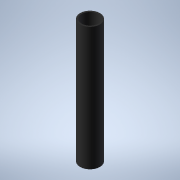
# Autodesk Inventor part: BZB-PDOWN
Saved by Autodesk Inventor 2021 (Build 250183000, 183)
## iProperties
Created: 2025-06-23
Part Number: BZB-PDOWN
Material: Generic
Catalog Web Link: www.cadenas.de
Description: base stand BZB-Accessories
Vendor: RNA
Document SubType Name: Modeling
Designer: psAdmin
Manufacturer: RNA
Mass: 179.196 g
Surface Area: 907.543 cm^2
Volume: 179.196 cm^3
Density: 1 g/cm^3
Appearance: PSOLRGB-175-175-175
Category: PARTsolutions
Company: RNA
Title: BZB-PDOWN
Author: Cadenas PARTsolutions
Comments: Accessories
PSOL_IDENT_0: {$CADENAS_DATA/23d-libs/rna/bunker/zubehoer/parts/bzb_profil_down.prj},166 {VTYP=3D},{NB=BZB-PDOWN},
PSOL_IDENT_1: {LINA=BZB-PDOWN},{NN=base stand BZB},{DATE=06.06.2017 07:14:33},{GEOMDATE=01.02.2017 10:27:25},{VERS
PSOL_IDENT_2: ION=},{LINEID=10},{WBVAR=},{WBNUMERIC=}  {NB=BZB-PDOWN},{LINA=BZB-PDOWN},{KT=DUMMY},{IDNR=BZB-PDOWN}
NB: BZB-PDOWN
NN: base stand BZB
NT: Accessories
NBSYN: $IDNR.
LINA: BZB-PDOWN
CATALOG: Rhein-Nadel-Automation
IDNR: BZB-PDOWN
SUPPLIER: RNA
ARTICLENO: BZB-PDOWN
BOMINFO: BZB-PDOWN
CREATOR: CADENAS GmbH
Autodesk Inventor part; units mm, degrees
sketch "Sketch_1" plane through (0, 0, 0) normal (0, 1, 0) x (-1, 0, 0)
  circle A0 centre (0, 0) radius 25
  circle A1 centre (0, 0) radius 21
  constraints: 2 centre point
extrude "Extrusion1" add sketch "Sketch_1" along normal blind 310
ref_plane "S1_DOWN_XY" through (0, 0, 0) normal (0, 1, 0) x (1, 0, 0)
ref_plane "S1_DOWN_YZ" through (0, 0, 0) normal (1, 0, 0) x (0, 0, -1)
ref_plane "S1_DOWN_ZX" through (0, 0, 0) normal (0, 0, -1) x (0, 1, 0)
ref_plane "S1_UP_XY" through (0, 310, 0) normal (0, -1, 0) x (1, 0, 0)
ref_plane "S1_UP_YZ" through (0, 310, 0) normal (1, 0, 0) x (0, 0, 1)
ref_plane "S1_UP_ZX" through (0, 310, 0) normal (0, 0, 1) x (0, -1, 0)
body "Solid1"
